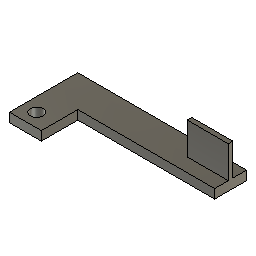
Z Flag (Autodesk Fusion 360 design; units mm, degrees)
Autodesk Fusion 360 part; units mm, degrees
sketch "Sketch1" plane through (0, 0, 0) normal (0, 0, 1) x (1, 0, 0)
  line L0 (16.5, -3.5) -> (-16.5, -3.5)
  line L1 (-16.5, -3.5) -> (-16.5, 3.5)
  line L2 (-16.5, 3.5) -> (16.5, 3.5)
  line L3 (16.5, 3.5) -> (16.5, -3.5)
  line L4 (16.5, -3.5) -> (-16.5, 3.5) construction
  line L5 (-16.5, -3.5) -> (16.5, 3.5) construction
  circle A0 centre (-13.5, -8.5) radius 1.4
  line L6 (-16.5, 3.5) -> (-9.5, 3.5)
  line L7 (-9.5, 3.5) -> (-9.5, -11.5)
  line L8 (-9.5, -11.5) -> (-16.5, -11.5)
  line L9 (-16.5, -11.5) -> (-16.5, 3.5)
  dimension "d1" = 33
  dimension "d2" = 7
  dimension "d3" = 2.8
  dimension "d4" = 3
  dimension "d16" = 15
  dimension "d17" = 3
  dimension "d18" = 7
  constraint horizontal L0
  constraint perpendicular L0 L1
  constraint parallel L0 L2
  constraint parallel L1 L3
  constraint coincident L4 origin
  constraint coincident L5 origin
  constraint horizontal L6
  constraint vertical L7
  constraint horizontal L8
  constraint vertical L9
  measures "d1" distance of L1.end L2.end
  measures "d2" distance of L0.end L1.end
  measures "d3" diameter of A0
  measures "d4" distance of L1 A0.centre
  measures "d16" distance of L1.end L8.end
  measures "d17" distance of A0.centre L8
  measures "d18" distance of L7 L9
extrude "Extrude1" add sketch "Sketch1" along normal blind 2
sketch "Sketch2" plane through (16.5, 0, 0) normal (1, 0, 0) x (0, 1, 0)
  line L0 (-3.5, 0) -> (3.5, 0)
  line L1 (3.5, 0) -> (3.5, 2)
  line L2 (3.5, 2) -> (-3.5, 2)
  line L3 (-3.5, 2) -> (-3.5, 0)
  line L4 (0, 2) -> (0.5, 2)
  line L5 (0.5, 2) -> (0.5, 12)
  line L6 (0.5, 12) -> (0, 12)
  line L7 (0, 12) -> (0, 2)
  line L8 (0, 12) -> (-0.5, 12)
  line L9 (-0.5, 12) -> (-0.5, 2)
  line L10 (-0.5, 2) -> (0, 2)
  line L11 (0, 2) -> (0, 12)
  dimension "d7" = 0.5
  dimension "d8" = 10
  dimension "d9" = 0.5
  constraint horizontal L4
  constraint vertical L5
  constraint horizontal L6
  constraint vertical L7
  constraint midpoint L2 L4.start
  constraint horizontal L8
  constraint vertical L9
  constraint horizontal L10
  constraint vertical L11
  measures "d7" distance of L4.start L4.end
  measures "d8" distance of L4.start L6.end
  measures "d9" distance of L6.end L8.end
extrude "Extrude2" add sketch "Sketch2" against normal blind 5 contours L2 L7 L8 L9 L10 L11 | L2 L4 L5 L6 L7 L11
extrude "Extrude3" add 1 faces at (16.5, 0.1667, 0.6667) along direction (1, 0, 0) blind 4
extrude "Extrude4" cut 1 faces at (17.5, -0.1667, 12) along direction (0, 0, -1) blind 3
equation "d1 = 25 mm + 8 mm"
